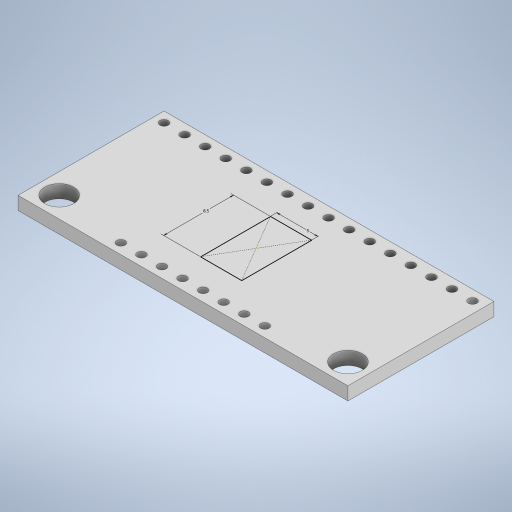
# Autodesk Inventor part: HW-178
Saved by Autodesk Inventor 2023.1 (Build 271208000, 208)
## iProperties
Created: 2022-07-25
Part Number: HW-178
Material: Generic
Document SubType Name: Modeling
Designer: fraaw
Density: 1 g/cm^3
Appearance: Default
Author: fraaw
Autodesk Inventor part; units mm, degrees
ref_plane "YZ Plane" through (0, 0, 0) normal (1, 0, 0) x (0, 1, 0)
ref_plane "XZ Plane" through (0, 0, 0) normal (0, 1, 0) x (-1, 0, 0)
ref_plane "XY Plane" through (0, 0, 0) normal (0, 0, 1) x (1, 0, 0)
sketch "Sketch1" plane through (0, 0, 0) normal (0, 1, 0) x (-1, 0, 0)
  line L0 (-20.05, 8.875) -> (20.05, 8.875)
  line L1 (20.05, 8.875) -> (20.05, -8.875)
  line L2 (20.05, -8.875) -> (-20.05, -8.875)
  line L3 (-20.05, -8.875) -> (-20.05, 8.875)
  line L4 (-20.05, 8.875) -> (20.05, -8.875) construction
  line L5 (20.05, 8.875) -> (-20.05, -8.875) construction
  point P0 (0, 0)
  dimension "d0" = 40
  dimension "d1" = 18
  constraints: 12 end point, 2 midpoint, 2 parallel, 1 horizontal, 1 perpendicular
extrude "Extrusion1" add sketch "Sketch1" along normal blind 1.6
sketch "Sketch2" plane through (0, 1.6, 0) normal (0, 1, 0) x (1, 0, 0)
  line L0 (-2.5, -4.25) -> (2.5, -4.25)
  line L1 (2.5, -4.25) -> (2.5, 4.25)
  line L2 (2.5, 4.25) -> (-2.5, 4.25)
  line L3 (-2.5, 4.25) -> (-2.5, -4.25)
  line L4 (-2.5, -4.25) -> (2.5, 4.25) construction
  line L5 (2.5, -4.25) -> (-2.5, 4.25) construction
  point P0 (0, 0)
  dimension "d7" = 5
  dimension "d8" = 8.5
  constraints: 12 end point, 2 midpoint, 2 parallel, 1 horizontal, 1 perpendicular
  measures "d7" distance of L1.end L2.end
  measures "d8" distance of L2.end L0.start
sketch "Sketch3" plane through (0, 1.6, 0) normal (0, 1, 0) x (1, 0, 0)
  circle A0 centre (-18.8, 7.625) radius 0.5
  line L0 (20.05, 8.875) -> (-20.05, 8.875) projected
  line L1 (-20.05, 8.875) -> (-20.05, -8.875) projected
  circle A1 centre (-16.3, 7.625) radius 0.5
  circle A2 centre (-13.8, 7.625) radius 0.5
  circle A3 centre (-11.3, 7.625) radius 0.5
  circle A4 centre (-8.8, 7.625) radius 0.5
  circle A5 centre (-6.3, 7.625) radius 0.5
  circle A6 centre (-3.8, 7.625) radius 0.5
  circle A7 centre (-1.3, 7.625) radius 0.5
  circle A8 centre (1.2, 7.625) radius 0.5
  circle A9 centre (3.7, 7.625) radius 0.5
  circle A10 centre (6.2, 7.625) radius 0.5
  circle A11 centre (8.7, 7.625) radius 0.5
  circle A12 centre (11.2, 7.625) radius 0.5
  circle A13 centre (13.7, 7.625) radius 0.5
  circle A14 centre (16.2, 7.625) radius 0.5
  circle A15 centre (18.7, 7.625) radius 0.5
  line L2 (-20.05, 0) -> (20.05, 0) construction
  line L3 (20.05, -8.875) -> (20.05, 8.875) construction
  circle A16 centre (-8.8, -7.625) radius 0.5
  circle A17 centre (-6.3, -7.625) radius 0.5
  circle A18 centre (-3.8, -7.625) radius 0.5
  circle A19 centre (-1.3, -7.625) radius 0.5
  circle A20 centre (1.2, -7.625) radius 0.5
  circle A21 centre (3.7, -7.625) radius 0.5
  circle A22 centre (6.2, -7.625) radius 0.5
  circle A23 centre (8.7, -7.625) radius 0.5
  circle A24 centre (-17.55, -6.375) radius 1.75
  line L4 (-20.05, -8.875) -> (20.05, -8.875) projected
  line L5 (0, 8.875) -> (0, -8.875) construction
  circle A25 centre (17.55, -6.375) radius 1.75
  point P0 (0, 0)
  dimension "d9" = 1
  dimension "d10" = 1.25
  dimension "d11" = 1.25
  dimension "d14" = 2.5
  dimension "d21" = 3.5
  dimension "d22" = 2.5
  dimension "d23" = 2.5
  constraints: 26 centre point, 9 symmetric about line, 4 end point, 4 midpoint, 1 horizontal, 39 other
  measures "d9" diameter of A0
  measures "d10" distance from line of L0 A0.centre
  measures "d11" distance from line of L1 A0.centre
  measures "d14" distance of A0.centre A1.centre
  measures "d21" diameter of A24
  measures "d22" distance from line of L1 A24.centre
  measures "d23" distance from line of L4 A24.centre
extrude "Extrusion2" cut sketch "Sketch3" against normal through all
body "Solid1"
